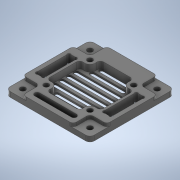
# Autodesk Inventor part: Camera_root_frame
Saved by Autodesk Inventor 2020.4 (Build 244396000, 396)
## iProperties
Created: 2021-12-31
Part Number: Camera_root_frame
Material: アセタール樹脂、黒
Document SubType Name: Modeling
Designer: Masato Kubotera
Density: 1.425 g/cm^3
Appearance: 滑らか - 黒
Description: POM T5
Mass: 8.05802 g
Surface Area: 52.0269 cm^2
Volume: 5.65475 cm^3
Author: Masato Kubotera
Autodesk Inventor part; units mm, degrees
ref_plane "YZ Plane" through (0, 0, 0) normal (1, 0, 0) x (0, 1, 0)
ref_plane "XZ Plane" through (0, 0, 0) normal (0, 1, 0) x (-1, 0, 0)
ref_plane "XY Plane" through (0, 0, 0) normal (0, 0, 1) x (1, 0, 0)
derived "KBCR-S08MM.ipt"
sketch "スケッチ1" plane through (0, 0, 0) normal (0, 0, 1) x (1, 0, 0)
  line L0 (14, 16) -> (-14, 16) construction
  line L1 (-16, 14) -> (-16, -14) construction
  line L2 (-14, -16) -> (14, -16) construction
  line L3 (16, -14) -> (16, 14) construction
  line L4 (16, 16) -> (-16, -16) construction
  line L5 (-16, 16) -> (16, -16) construction
  line L6 (-13, 13) -> (13, 13) construction
  line L7 (13, 13) -> (13, -13) construction
  line L8 (13, -13) -> (-13, -13) construction
  line L9 (-13, -13) -> (-13, 13) construction
  line L10 (-13, 13) -> (13, -13) construction
  line L11 (13, 13) -> (-13, -13) construction
  circle A0 centre (-13, -13) radius 1.1 construction
  line L12 (-16, 0) -> (16, 0) construction
  line L13 (0, 16) -> (0, -16) construction
  circle A1 centre (-13, 13) radius 1.1 construction
  circle A2 centre (13, 13) radius 1.1 construction
  circle A3 centre (13, -13) radius 1.1 construction
  circle A4 centre (-13, -13) radius 2 construction
  circle A5 centre (-13, 13) radius 2 construction
  circle A6 centre (13, -13) radius 2 construction
  circle A7 centre (13, 13) radius 2 construction
  circle A8 centre (0, 0) radius 7.5 construction
  circle A9 centre (-5.5, -9) radius 1.1 construction
  circle A10 centre (-5.5, -9) radius 2 construction
  line L14 (-7.5, -9) -> (-7.5, 7.5) construction
  line L15 (-7.5, 7.5) -> (3.5, 7.5) construction
  line L16 (-3.5, -9) -> (-3.5, -7.5) construction
  circle A11 centre (5.5, 9) radius 2 construction
  line L17 (3.5, 9) -> (3.5, 7.5) construction
  circle A12 centre (5.5, 9) radius 1.1 construction
  line L18 (7.5, 9) -> (7.5, -7.5) construction
  line L19 (7.5, -7.5) -> (-3.5, -7.5) construction
  arc A13 (-16, -14) -> (-14, -16) centre (-14, -14) ccw construction
  arc A14 (14, -16) -> (16, -14) centre (14, -14) ccw construction
  arc A15 (16, 14) -> (14, 16) centre (14, 14) ccw construction
  arc A16 (-14, 16) -> (-16, 14) centre (-14, 14) ccw construction
  line L20 (16, -11.1) -> (15, -11.1) construction
  line L21 (15, -11.1) -> (15, 11.1) construction
  line L22 (16, 11.1) -> (15, 11.1) construction
sketch "スケッチ2" plane through (0, 0, 0) normal (0, 0, 1) x (1, 0, 0)
  line L0 (-22.5, 25) -> (22.5, 25)
  line L1 (25, 22.5) -> (25, -22.5)
  line L2 (22.5, -25) -> (-22.5, -25)
  line L3 (-25, -22.5) -> (-25, 22.5)
  line L4 (-25, 25) -> (25, -25) construction
  line L5 (25, 25) -> (-25, -25) construction
  arc A0 (-22.5, 25) -> (-25, 22.5) centre (-22.5, 22.5) ccw
  arc A1 (-25, -22.5) -> (-22.5, -25) centre (-22.5, -22.5) ccw
  arc A2 (22.5, -25) -> (25, -22.5) centre (22.5, -22.5) ccw
  arc A3 (25, 22.5) -> (22.5, 25) centre (22.5, 22.5) ccw
  line L6 (-25, -22.5) -> (25, -22.5) construction
  line L7 (25, -22.5) -> (25, -17.5)
  line L8 (25, -17.5) -> (-25, -17.5) construction
  line L9 (-25, -17.5) -> (-25, -22.5) construction
  line L10 (-25, -22.5) -> (25, -17.5) construction
  line L11 (25, -22.5) -> (-25, -17.5) construction
  line L12 (-25, -20) -> (25, -20) construction
  line L13 (0, 16) -> (0, -16) construction
  circle A4 centre (-20, -20) radius 1.6
  circle A5 centre (20, -20) radius 1.6
  line L14 (-16, 0) -> (16, 0) construction
  circle A6 centre (-20, 20) radius 1.6
  circle A7 centre (20, 20) radius 1.6
  circle A8 centre (-5.5, -9) radius 2 construction
  circle A9 centre (13, 13) radius 1.1 projected
  circle A10 centre (13, -13) radius 1.1 projected
  circle A11 centre (-13, -13) radius 1.1 projected
  circle A12 centre (-13, 13) radius 1.1 projected
  circle A13 centre (-13, -13) radius 1.55
  circle A14 centre (13, -13) radius 1.55
  circle A15 centre (13, 13) radius 1.55
  circle A16 centre (-13, 13) radius 1.55
  line L15 (-14, -16) -> (14, -16) projected
  line L16 (-16, 14) -> (-16, -14) projected
  line L17 (-16, -7.8461) -> (-16, 0)
  line L18 (0, -16) -> (-7.8461, -16)
  arc A17 (-9.8095, -13.619) -> (-13.619, -9.8095) centre (-13, -13) ccw
  arc A18 (-9.8095, -13.619) -> (-7.8461, -16) centre (-7.8461, -14) ccw
  arc A19 (-16, -7.8461) -> (-13.619, -9.8095) centre (-14, -7.8461) ccw
  line L19 (-16, 7.8461) -> (-16, 0)
  line L20 (0, 16) -> (-7.8461, 16)
  arc A20 (-13.619, 9.8095) -> (-9.8095, 13.619) centre (-13, 13) ccw
  arc A21 (-7.8461, 16) -> (-9.8095, 13.619) centre (-7.8461, 14) ccw
  arc A22 (-13.619, 9.8095) -> (-16, 7.8461) centre (-14, 7.8461) ccw
  line L21 (16, -7.8461) -> (16, 0)
  line L22 (0, -16) -> (7.8461, -16)
  arc A23 (13.619, -9.8095) -> (9.8095, -13.619) centre (13, -13) ccw
  arc A24 (7.8461, -16) -> (9.8095, -13.619) centre (7.8461, -14) ccw
  arc A25 (13.619, -9.8095) -> (16, -7.8461) centre (14, -7.8461) ccw
  arc A26 (16, 7.8461) -> (13.619, 9.8095) centre (14, 7.8461) ccw
  arc A27 (9.8095, 13.619) -> (7.8461, 16) centre (7.8461, 14) ccw
  line L23 (16, 7.8461) -> (16, 0)
  line L24 (0, 16) -> (7.8461, 16)
  arc A28 (9.8095, 13.619) -> (13.619, 9.8095) centre (13, 13) ccw
  line L25 (-10, -22.5) -> (10, -22.5) construction
  line L26 (10, -22.5) -> (10, -17.5) construction
  line L27 (10, -17.5) -> (-10, -17.5) construction
  line L28 (-10, -17.5) -> (-10, -22.5) construction
  line L29 (-10, -22.5) -> (10, -17.5) construction
  line L30 (10, -22.5) -> (-10, -17.5) construction
  line L31 (-8.5651, -22.55) -> (8.5651, -22.55)
  line L32 (8.5651, -17.45) -> (-8.5651, -17.45)
  arc A29 (-10.05, -21.0651) -> (-8.5651, -22.55) centre (-9.3075, -21.8075) ccw
  arc A30 (-8.5651, -17.45) -> (-10.05, -18.9349) centre (-9.3075, -18.1925) ccw
  arc A31 (8.5651, -22.55) -> (10.05, -21.0651) centre (9.3075, -21.8075) ccw
  arc A32 (10.05, -18.9349) -> (8.5651, -17.45) centre (9.3075, -18.1925) ccw
  line L33 (-10.05, -22.5) -> (-10.05, -22.55)
  line L34 (-10.05, -18.9349) -> (-10.05, -21.0651)
  line L35 (10.05, -21.0651) -> (10.05, -18.9349)
  line L36 (-8.5651, 22.55) -> (8.5651, 22.55)
  line L37 (8.5651, 17.45) -> (-8.5651, 17.45)
  arc A33 (-8.5651, 22.55) -> (-10.05, 21.0651) centre (-9.3075, 21.8075) ccw
  arc A34 (-10.05, 18.9349) -> (-8.5651, 17.45) centre (-9.3075, 18.1925) ccw
  arc A35 (8.5651, 17.45) -> (10.05, 18.9349) centre (9.3075, 18.1925) ccw
  arc A36 (10.05, 21.0651) -> (8.5651, 22.55) centre (9.3075, 21.8075) ccw
  line L38 (-10.05, 18.9349) -> (-10.05, 21.0651)
  line L39 (10.05, 21.0651) -> (10.05, 18.9349)
  line L40 (19, -11) -> (22, -11) construction
  line L41 (22, -11) -> (22, 11)
  line L42 (22, 11) -> (19, 11) construction
  line L43 (19, 11) -> (19, -11)
  line L44 (19, -11) -> (22, 11) construction
  line L45 (22, -11) -> (19, 11) construction
  arc A37 (19, -11) -> (22, -11) centre (20.5, -11) ccw
  arc A38 (22, 11) -> (19, 11) centre (20.5, 11) ccw
  arc A39 (-15, -17) -> (-15.5858, -15.5858) centre (-17, -17) ccw
  line L46 (-15, -17) -> (-15, -23)
  arc A40 (-14.9998, -22.9729) -> (-13, -25) centre (-13, -23) ccw
  arc A41 (-15.5858, -15.5858) -> (-17, -15) centre (-17, -17) ccw
  line L47 (-17, -15) -> (-23, -15)
  arc A42 (-25, -13) -> (-22.9729, -14.9998) centre (-23, -13) ccw
  arc A43 (-15.5858, 15.5858) -> (-15, 17) centre (-17, 17) ccw
  line L48 (-15, 17) -> (-15, 23)
  arc A44 (-13, 25) -> (-14.9998, 22.9729) centre (-13, 23) ccw
  arc A45 (-17, 15) -> (-15.5858, 15.5858) centre (-17, 17) ccw
  line L49 (-17, 15) -> (-23, 15)
  arc A46 (-22.9729, 14.9998) -> (-25, 13) centre (-23, 13) ccw
  arc A47 (15.5858, -15.5858) -> (15, -17) centre (17, -17) ccw
  line L50 (15, -17) -> (15, -23)
  arc A48 (13, -25) -> (14.9998, -22.9729) centre (13, -23) ccw
  arc A49 (17, -15) -> (15.5858, -15.5858) centre (17, -17) ccw
  line L51 (17, -15) -> (23, -15)
  arc A50 (22.9729, -14.9998) -> (25, -13) centre (23, -13) ccw
  arc A51 (25, 13) -> (22.9729, 14.9998) centre (23, 13) ccw
  line L52 (17, 15) -> (23, 15)
  arc A52 (15.5858, 15.5858) -> (17, 15) centre (17, 17) ccw
  arc A53 (15, 17) -> (15.5858, 15.5858) centre (17, 17) ccw
  line L53 (15, 17) -> (15, 23)
  arc A54 (14.9998, 22.9729) -> (13, 25) centre (13, 23) ccw
  line L54 (20.5, -12.5) -> (20.5, 12.5) construction
  line L55 (-16, -7.8461) -> (-13.5, -7.8461) construction
  line L56 (-13.5, -7.8461) -> (-13.5, 7.8461)
  line L57 (-13.5, 7.8461) -> (-16, 7.8461) construction
  line L58 (-16, 7.8461) -> (-16, -7.8461)
  line L59 (-16, -7.8461) -> (-13.5, 7.8461) construction
  line L60 (-13.5, -7.8461) -> (-16, 7.8461) construction
  arc A55 (-16, -7.8461) -> (-13.5, -7.8461) centre (-14.75, -7.8461) ccw
  arc A56 (-13.5, 7.8461) -> (-16, 7.8461) centre (-14.75, 7.8461) ccw
  line L61 (-11.7857, -9.2347) -> (-9.2857, -9.2347) construction
  line L62 (-9.2857, -9.2347) -> (-9.2857, 9.2347)
  line L63 (-9.2857, 9.2347) -> (-11.7857, 9.2347) construction
  line L64 (-11.7857, 9.2347) -> (-11.7857, -9.2347)
  line L65 (-11.7857, -9.2347) -> (-9.2857, 9.2347) construction
  line L66 (-9.2857, -9.2347) -> (-11.7857, 9.2347) construction
  arc A57 (-11.7857, -9.2347) -> (-9.2857, -9.2347) centre (-10.5357, -9.2347) ccw
  arc A58 (-9.2857, 9.2347) -> (-11.7857, 9.2347) centre (-10.5357, 9.2347) ccw
  line L67 (13.5, -7.8461) -> (13.5, 7.8461)
  line L68 (16, 7.8461) -> (16, -7.8461)
  arc A59 (13.5, -7.8461) -> (16, -7.8461) centre (14.75, -7.8461) ccw
  arc A60 (16, 7.8461) -> (13.5, 7.8461) centre (14.75, 7.8461) ccw
  arc A61 (9.2857, -9.2347) -> (11.7857, -9.2347) centre (10.5357, -9.2347) ccw
  line L69 (9.2857, -9.2347) -> (9.2857, 9.2347)
  line L70 (11.7857, 9.2347) -> (11.7857, -9.2347)
  arc A62 (11.7857, 9.2347) -> (9.2857, 9.2347) centre (10.5357, 9.2347) ccw
  line L71 (-7.5714, -14.75) -> (-5.0714, -14.75) construction
  arc A63 (-7.5714, -14.75) -> (-5.0714, -14.75) centre (-6.3214, -14.75) ccw
  line L72 (-5.0714, -14.75) -> (-5.0714, 14.75)
  line L73 (-7.5714, -14.75) -> (-5.0714, 14.75) construction
  line L74 (-7.5714, 14.75) -> (-7.5714, -14.75)
  line L75 (-5.0714, -14.75) -> (-7.5714, 14.75) construction
  line L76 (-5.0714, 14.75) -> (-7.5714, 14.75) construction
  arc A64 (-5.0714, 14.75) -> (-7.5714, 14.75) centre (-6.3214, 14.75) ccw
  line L77 (-0.8571, -14.75) -> (-0.8571, 14.75)
  line L78 (-3.3571, -14.75) -> (-0.8571, 14.75) construction
  line L79 (-0.8571, -14.75) -> (-3.3571, 14.75) construction
  line L80 (-3.3571, 14.75) -> (-3.3571, -14.75)
  line L81 (-0.8571, 14.75) -> (-3.3571, 14.75) construction
  arc A65 (-0.8571, 14.75) -> (-3.3571, 14.75) centre (-2.1071, 14.75) ccw
  arc A66 (-3.3571, -14.75) -> (-0.8571, -14.75) centre (-2.1071, -14.75) ccw
  line L82 (-3.3571, -14.75) -> (-0.8571, -14.75) construction
  line L83 (16, 0) -> (-16, 0) construction
  line L84 (5.0714, -14.75) -> (5.0714, 14.75)
  line L85 (7.5714, -14.75) -> (5.0714, 14.75) construction
  line L86 (5.0714, -14.75) -> (7.5714, 14.75) construction
  line L87 (7.5714, 14.75) -> (7.5714, -14.75)
  line L88 (5.0714, 14.75) -> (7.5714, 14.75) construction
  arc A67 (7.5714, 14.75) -> (5.0714, 14.75) centre (6.3214, 14.75) ccw
  arc A68 (5.0714, -14.75) -> (7.5714, -14.75) centre (6.3214, -14.75) ccw
  line L89 (7.5714, -14.75) -> (5.0714, -14.75) construction
  line L90 (0.8571, -14.75) -> (0.8571, 14.75)
  line L91 (0.8571, -14.75) -> (3.3571, 14.75) construction
  line L92 (3.3571, -14.75) -> (0.8571, 14.75) construction
  line L93 (3.3571, 14.75) -> (3.3571, -14.75)
  arc A69 (0.8571, -14.75) -> (3.3571, -14.75) centre (2.1071, -14.75) ccw
  line L94 (3.3571, -14.75) -> (0.8571, -14.75) construction
  line L95 (0.8571, 14.75) -> (3.3571, 14.75) construction
  arc A70 (3.3571, 14.75) -> (0.8571, 14.75) centre (2.1071, 14.75) ccw
  point P0 (0, 0)
  point P1 (0, -20)
  point P2 (0, -20)
  point P3 (-16, -11.75)
  point P4 (-11.75, -16)
  point P5 (20.5, 0)
  point P6 (20.5, 0)
  point P7 (-16, -7.8461)
  point P8 (-16, 7.8461)
  point P9 (7.8461, -16)
  point P10 (13, -25)
  point P11 (25, -13)
  point P12 (25, 13)
  point P13 (13, 25)
  point P14 (-13, 25)
  point P15 (-25, 13)
  point P16 (-25, -13)
  point P17 (-14.75, 0)
  point P18 (-10.5357, 0)
  point P19 (-10.5357, 0)
  point P20 (-6.3214, 0)
  point P21 (-6.3214, 0)
  point P22 (-6.3214, 0)
  point P23 (30.5, 10)
  point P24 (-2.1071, 0)
  point P25 (-2.1071, 0)
  point P26 (-2.1071, 0)
  point P27 (5.5, -9)
  point P28 (6.3214, 0)
  point P29 (6.3214, 0)
  point P30 (6.3214, 0)
  point P31 (2.1071, 0)
  point P32 (2.1071, 0)
  point P33 (2.1071, 0)
  point P34 (6.3214, 16)
  point P35 (2.1071, 16)
  point P36 (3.3571, 14.75)
  point P37 (2.1071, -16)
  point P38 (6.3214, -16)
  point P39 (-2.1071, -16)
  point P40 (-2.1071, 16)
  point P41 (-6.3214, -16)
  point P42 (-3.3571, 14.75)
  point P43 (-6.3214, 16)
  point P44 (-11.2202, -10.2806)
  point P45 (-11.7857, 9.2347)
  point P46 (-11.2202, 10.2806)
  point P47 (-16, 7.8461)
  point P48 (7.5714, 14.75)
  point P49 (11.2202, -10.2806)
  point P50 (11.2202, 10.2806)
  point P51 (11.7857, 9.2347)
  point P52 (-7.5714, 14.75)
  dimension "d1" = 50
  dimension "d2" = 50
  dimension "d3" = 2.5
  dimension "d7" = 5
  dimension "d8" = 5
  dimension "d9" = 3.2
  dimension "d10" = 5
  dimension "d12" = 3.1
  dimension "d14" = 3.1
  dimension "d15" = 3.1
  dimension "d16" = 3.1
  dimension "d19" = 1.7
  dimension "d20" = 2
  dimension "d21" = 40
  dimension "d23" = 10
  dimension "d24" = 20
  dimension "d27" = 0.05
  dimension "d28" = 1.05
  dimension "d30" = 0.05
  dimension "d31" = 3
  dimension "d33" = 9
  dimension "d34" = 4.5
  dimension "d39" = 2
  dimension "d40" = 2
  dimension "d41" = 5
  dimension "d42" = 25
  dimension "d45" = 2.5
  dimension "d46" = 16
  dimension "d47" = 2.5
  dimension "d48" = 2.5
  dimension "d50" = 2.5
  dimension "d51" = 0.8571
  dimension "d55" = 1.7143
  dimension "d56" = 1.7143
  dimension "d57" = 1.7143
  constraints: 184 end point, 129 point on circle, 124 symmetric about line, 66 centre point, 38 midpoint, 35 point on line, 19 parallel, 19 tangent, 9 horizontal, 9 perpendicular, 5 coincident, 4 equal radius, 2 collinear, 1 vertical, 42 other
  measures "d1" distance of L4.end L5.end
  measures "d2" distance of L5.start L4.end
  measures "d3" radius of A0
  measures "d7" distance of L7.end L6.end
  measures "d8" distance from line of L5.end L12
  measures "d9" diameter of A4
  measures "d10" distance of L12.start A4.centre
  measures "d12" diameter of A13
  measures "d14" diameter of A14
  measures "d15" diameter of A15
  measures "d16" diameter of A16
  measures "d19" radial gap between concentric circles of A17 A13
  measures "d20" radius of A18
  measures "d21" distance of A6.centre A4.centre
  measures "d23" horizontal distance of L25.start A4.centre
  measures "d24" distance of L25.end L25.start
  measures "d27" distance between parallel lines of L31 L25
  measures "d28" radius of A29
  measures "d30" distance between parallel lines of L28 L34
  measures "d31" distance of L42.end L41.end
  measures "d33" distance from line of L1 L14.end
  measures "d34" distance of L14.end point (20.5, 0)
  measures "d39" radius of A40
  measures "d40" radius of A39
  measures "d41" horizontal distance of L46.end A4.centre
  measures "d42" distance of L54.start L54.end
  measures "d45" distance of L57.end L56.end
  measures "d46" distance of point (0, 0) L14.start
  measures "d47" distance of L64.start L62.end
  measures "d48" distance of L75.end L72.end
  measures "d50" distance of L79.end L77.end
  measures "d51" distance from line of L13 L77.start
  measures "d55" distance between parallel lines of L80 L72
  measures "d56" distance between parallel lines of L74 L62
  measures "d57" distance between parallel lines of L64 L56
extrude "押し出し1" add sketch "スケッチ2" along normal blind 5 contours L0 A54 L53 A53 A52 L52 A51 L1 A50 L51 A49 A47 L50 A48 L2 A40 L46 A39 A41 L47 A42 L3 A46 L49 A45 A43 L48 A44
extrude "押し出し2" add sketch "スケッチ2" along normal blind 1 contours A18 A17 A57 L62 A58 A20 A21 L20 A64 L74 A63 L15 | A63 L72 A64 L20 A65 L80 A66 L15 | A66 L77 A65 L20 L24 A70 L90 A69 L15 | A17 A19 A55 L56 A56 A22 A20 A58 L64 A57 | A69 L93 A70 L24 A67 L84 A68 L15 | A68 L87 A67 L24 A27 A28 A62 L69 A61 A23 A24 L15 | A61 L70 A62 A28 A26 A60 L67 A59 A25 A23
extrude "押し出し3" add sketch "スケッチ2" along normal blind 3 contours L0 A44 L48 A43 A45 L49 A46 L3 A0 | L0 A3 L1 A51 L52 A52 A53 L53 A54 | A42 L47 A41 A39 L46 A40 L2 A1 L3 | L1 A2 L2 A48 L50 A47 A49 L51 A50
equation "\"d14\" = d12"
equation "\"d15\" = d12"
equation "\"d16\" = d12"
equation "\"d27\" = d26"
equation "\"d34\" = 0.5 * d33"
equation "\"d40\" = d39"
equation "\"d41\" = d10"
equation "\"d26\" = 0.05"
